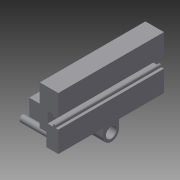
# Autodesk Inventor part: Karetka
Saved by Autodesk Inventor 2015 (Build 190159000, 159)
## iProperties
Created: 2016-04-08
Part Number: Karetka
Material: Generic
Document SubType Name: Modeling
Designer: Andreas
Density: 1 g/cm^3
Appearance: Default
Author: Andreas
Autodesk Inventor part; units mm, degrees
ref_plane "YZ Plane" through (0, 0, 0) normal (1, 0, 0) x (0, 1, 0)
ref_plane "XZ Plane" through (0, 0, 0) normal (0, 1, 0) x (-1, 0, 0)
ref_plane "XY Plane" through (0, 0, 0) normal (0, 0, 1) x (1, 0, 0)
sketch "Sketch1" plane through (0, 0, 0) normal (0, 1, 0) x (-1, 0, 0)
  line L0 (0, 0) -> (0, 8)
  line L1 (0, 8) -> (7, 8)
  line L2 (7, 8) -> (7, -12)
  line L3 (7, -12) -> (0, -12)
  line L4 (0, -12) -> (0, -4)
  line L5 (0, -4) -> (4, -4)
  line L6 (4, -4) -> (4, 0)
  line L7 (4, 0) -> (0, 0)
  dimension "d0" = 8
  dimension "d1" = 7
  dimension "d2" = 20
  dimension "d3" = 7
  dimension "d4" = 8
  dimension "d5" = 4
  dimension "d6" = 4
  constraints: 16 end point, 5 perpendicular, 2 vertical
  measures "d0" distance of L0.start L0.end
  measures "d1" distance of L0.end L1.end
  measures "d2" distance of L1.end L2.end
  measures "d3" distance of L2.end L3.end
  measures "d4" distance of L3.end L4.end
  measures "d5" distance of L4.end L5.end
  measures "d6" distance of L5.end L6.end
extrude "Extrusion1" add sketch "Sketch1" along normal blind 40
sketch "Sketch5" plane through (0, 0, 0) normal (0, -1, 0) x (1, 0, 0)
  line L0 (-1, -4) -> (-1, -3.5)
  line L1 (-1.5, -3) -> (-1.5, -3)
  line L2 (-2, -3.5) -> (-2, -4)
  line L3 (-2, -4) -> (-1, -4)
  line L4 (-1, -0.5) -> (-1, 0)
  line L5 (-1, 0) -> (-2, 0)
  line L6 (-2, 0) -> (-2, -0.5)
  line L7 (-1.5, -1) -> (-1.5, -1)
  arc A0 (-1.5, -3) -> (-2, -3.5) centre (-1.5, -3.5) ccw
  arc A1 (-1, -3.5) -> (-1.5, -3) centre (-1.5, -3.5) ccw
  arc A2 (-2, -0.5) -> (-1.5, -1) centre (-1.5, -0.5) ccw
  arc A3 (-1.5, -1) -> (-1, -0.5) centre (-1.5, -0.5) ccw
  point P0 (0, 0)
  point P1 (-1, -3)
  point P2 (-2, -3)
  point P3 (-1, -1)
  point P4 (-2, -1)
  point P5 (-1.5, 0)
  point P6 (-1.5, -4)
  point P7 (0, -4)
  dimension "d35" = 1
  dimension "d36" = 1
  dimension "d37" = 1
  dimension "d38" = 1
  dimension "d39" = 1
  dimension "d40" = 1
  dimension "d41" = 0.5
  dimension "d42" = 1
  dimension "d43" = 1
  constraints: 16 end point, 10 point on line, 8 point on circle, 8 tangent, 4 centre point, 3 equal radius, 3 perpendicular, 2 horizontal alignment, 2 midpoint, 1 horizontal, 1 vertical
  measures "d35" distance of L0.start point (-1, -3)
  measures "d36" distance of point (-1, -3) point (-2, -3)
  measures "d37" distance of point (-2, -3) L2.end
  measures "d38" distance of point (-1, -1) L4.end
  measures "d39" distance of L4.end L5.end
  measures "d40" distance of L5.end point (-2, -1)
  measures "d41" radius of A0
  measures "d42" distance from line of point (0, -4) L0
  measures "d43" horizontal distance of point (0, 0) L4.start
extrude "Extrusion2" add sketch "Sketch5" against normal blind 40
sketch "Sketch7" plane through (-7, 0, -12) normal (-1, 0, 0) x (0, 0, 1)
  line L0 (8, 0) -> (8, 5)
  line L1 (8, 0) -> (8, 40) projected
  line L2 (8, 5) -> (0, 5)
  line L3 (0, 0) -> (0, 40) projected
  line L4 (0, 35) -> (8, 35)
  line L5 (8, 40) -> (8, 0)
  line L6 (0, 0) -> (8, 0) projected
  point P0 (12, 0)
  dimension "d51" = 5
  constraints: 8 end point, 4 point on line, 2 perpendicular, 1 parallel
  measures "d51" distance of L0.start L0.end
extrude "Extrusion4" add sketch "Sketch7" along normal blind 9
sketch "Sketch8" plane through (-16, 0, -12) normal (-1, 0, 0) x (0, 0, 1)
  line L0 (0, 40) -> (20, 40) projected
  line L1 (20, 0) -> (8, 0) projected
  line L2 (0, 40) -> (0, 23)
  line L3 (0, 0) -> (0, 40) projected
  line L4 (0, 23) -> (-3, 23)
  line L5 (0, 0) -> (0, 17)
  line L6 (0, 17) -> (-3, 17)
  arc A0 (-3, 23) -> (-3, 17) centre (-3, 20) ccw
  circle A1 centre (-3, 20) radius 2
  point P0 (12, 0)
  dimension "d56" = 40
  dimension "d57" = 17
  dimension "d58" = 3
  dimension "d59" = 17
  dimension "d60" = 3
  dimension "d61" = 4
  constraints: 8 end point, 2 centre point, 2 perpendicular, 2 point on circle, 2 point on line, 1 coincident, 1 tangent
  measures "d56" distance between parallel lines of L0 L1
  measures "d57" distance of L0.start L2.end
  measures "d58" distance of L2.end L4.end
  measures "d59" distance of L3.start L5.end
  measures "d60" distance of L5.end L6.end
  measures "d61" diameter of A1
extrude "Extrusion5" add sketch "Sketch8" against normal blind 16
sketch "Sketch10" plane through (-7, 0, -12) normal (-1, 0, 0) x (0, 0, 1)
  line L0 (0, 0) -> (5, 0)
  line L1 (5, 0) -> (5, 5)
  line L2 (5, 5) -> (0, 5)
  line L3 (0, 5) -> (0, 0)
  line L4 (0, 35) -> (5, 35)
  line L5 (5, 35) -> (5, 40)
  line L6 (5, 40) -> (0, 40)
  line L7 (0, 40) -> (0, 35)
  point P0 (12, 0)
  dimension "d64" = 5
  dimension "d65" = 5
  dimension "d66" = 5
  dimension "d67" = 5
  constraints: 16 end point, 4 parallel, 2 horizontal, 2 perpendicular
  measures "d64" distance of L2.end L1.end
  measures "d65" distance of L1.end L0.end
  measures "d66" distance of L6.end L5.end
  measures "d67" distance of L5.end L4.end
extrude "Extrusion6" cut sketch "Sketch10" against normal blind 2.5
sketch "Sketch11" plane through (-16, 0, -12) normal (-1, 0, 0) x (0, 0, 1)
  line L0 (0, 0) -> (8, 0)
  line L1 (8, 0) -> (8, 5)
  line L2 (8, 5) -> (0, 5)
  line L3 (0, 5) -> (0, 0)
  point P0 (12, 0)
  dimension "d70" = 8
  dimension "d71" = 5
  constraints: 8 end point, 2 parallel, 1 coincident, 1 horizontal, 1 perpendicular
  measures "d70" distance of L2.end L1.end
  measures "d71" distance of L1.end L0.end
extrude "Extrusion7" cut sketch "Sketch11" against normal blind 9
sketch "Sketch12" plane through (-4.5, 0, -12) normal (-1, 0, 0) x (0, 0, 1)
  circle A0 centre (2.5, 2.5) radius 1.25
  circle A1 centre (2.5, 37.5) radius 1.25
  point P0 (12, 0)
  dimension "d74" = 2.5
  dimension "d75" = 2.5
  constraints: 2 centre point
  measures "d74" diameter of A0
  measures "d75" diameter of A1
extrude "Extrusion8" add sketch "Sketch12" along normal blind 11.5
sketch "Sketch4" plane through (-4, 0, 0) normal (1, 0, 0) x (0, 0, -1)
  point P0 (5, 30)
  point P1 (5, 10)
body "Solid1"
